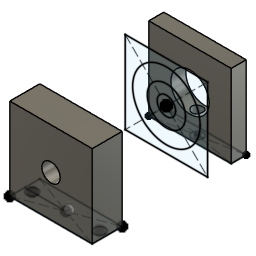
ThumbBrackets v2 (Autodesk Fusion 360 design; units mm, degrees)
Autodesk Fusion 360 part; units mm, degrees
sketch "Sketch2" plane through (0, 0, 0) normal (0, 0, 1) x (1, 0, 0)
  circle A0 centre (0, 0) radius 2.45
  line L0 (11, 11) -> (-11, 11)
  line L1 (-11, 11) -> (-11, -11)
  line L2 (-11, -11) -> (11, -11)
  line L3 (11, -11) -> (11, 11)
  line L4 (11, 11) -> (-11, -11) construction
  line L5 (-11, 11) -> (11, -11) construction
  circle A1 centre (0, 0) radius 9
  circle A2 centre (0, 0) radius 5.1
  dimension "d17" = 4.9
  dimension "d18" = 22
  dimension "d90" = 18
  dimension "d104" = 10.2
  dimension "d121" = 22
  constraint coincident A0.centre A1.centre
  constraint horizontal L0
  constraint perpendicular L0 L1
  constraint parallel L0 L2
  constraint parallel L1 L3
  constraint coincident L4 A0.centre
  constraint coincident L5 A0.centre
  constraint concentric A0 A1
  measures "d17" diameter of A0
  measures "d18" distance of L1.end L2.end
  measures "d90" diameter of A1
  measures "d104" diameter of A2
  measures "d121" distance of L0.start L2.end
extrude "Extrude3" add sketch "Sketch2" against normal blind 4 from surface at -6.3 contours A0 | L0 L1 L2 L3 | A1 | A2 makes body 1
extrude "Extrude4" add sketch "Sketch2" along normal blind 4 from surface at 22.8 separate body contours L0 L1 L2 L3 makes body 2
extrude "Extrude5" add sketch "Sketch2" along normal blind 4 from surface at 26.8 contours L0 L1 L2 L3 | A1 | A2 bodies 2
sketch "Sketch7" plane through (0, -11, 0) normal (0, -1, 0) x (1, 0, 0)
  line L0 (-11, 22.8) -> (11, 22.8)
  line L1 (11, 22.8) -> (11, 30.8)
  line L2 (11, 30.8) -> (-11, 30.8)
  line L3 (-11, 30.8) -> (-11, 22.8)
  line L4 (11, 22.8) -> (-11, 22.8)
  line L5 (-11, 22.8) -> (-11, 30.8)
  line L6 (-11, 30.8) -> (11, 30.8)
  line L7 (11, 30.8) -> (11, 22.8)
  line L8 (11, 30.8) -> (-11, 22.8) construction
  line L9 (-11, 30.8) -> (11, 22.8) construction
  line L10 (0, 26.8) -> (-11, 26.8)
  circle A0 centre (-9, 26.8) radius 1.425
  line L11 (0, 26.8) -> (0, 26)
  circle A1 centre (9, 26.8) radius 1.425
  point P0 (0, 26.8)
  dimension "d98" = 2.85
  dimension "d99" = 9
  constraint horizontal L4
  constraint vertical L5
  constraint horizontal L6
  constraint vertical L7
  constraint coincident L2.end L3.start
  constraint coincident L0.end L1.start
  constraint midpoint L8 P0
  constraint midpoint L5 L10.end
  constraint coincident L10 A0.centre
  constraint coincident P0 L10.start
  constraint perpendicular L10 L11
  constraint symmetric A0 L11 A1
  measures "d98" diameter of A0
  measures "d99" distance of A0.centre P0
sketch "Sketch8" plane through (0, -11, 0) normal (0, -1, 0) x (1, 0, 0)
  line L0 (11, -6.3) -> (-11, -6.3)
  line L1 (-11, -6.3) -> (-11, -10.3)
  line L2 (-11, -10.3) -> (11, -10.3)
  line L3 (11, -10.3) -> (11, -6.3)
  line L4 (11, -10.3) -> (-11, -10.3)
  line L5 (-11, -10.3) -> (-11, -6.3)
  line L6 (-11, -6.3) -> (11, -6.3)
  line L7 (11, -6.3) -> (11, -10.3)
  line L8 (11, -10.3) -> (-11, -6.3) construction
  line L9 (11, -6.3) -> (-11, -10.3) construction
  circle A0 centre (0, -8.3) radius 1.425
  dimension "d72" = 2.85
  constraint horizontal L4
  constraint vertical L5
  constraint horizontal L6
  constraint vertical L7
  constraint coincident L0.end L1.start
  constraint coincident L2.end L3.start
  constraint midpoint L9 A0.centre
  measures "d72" diameter of A0
extrude "Extrude9" cut sketch "Sketch7" sketch "Sketch8" against normal blind 7 contours L10 A0 | L10 A0 | A1 of sketch 2 contours A0 bodies 1 2
extrude "Extrude11" cut sketch "Sketch2" against normal blind 10.5 contours A0 | A2 bodies 1
equation "d19 = -6 mm - 0.3 mm"
equation "d22 = 22.5 mm + 0.3 mm"
equation "d26 = 22.5 mm + 0.3 mm + 4 mm"
